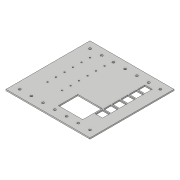
# Autodesk Inventor part: panel
Saved by Autodesk Inventor 2017 (Build 210142000, 142)
## iProperties
Created: 2016-07-20
Part Number: panel
Material: Generic
Document SubType Name: Modeling
Designer: Zuhra Abdurashidova
Density: 1 g/cm^3
Appearance: Default
Author: Zuhra Abdurashidova
Autodesk Inventor part; units mm, degrees
ref_plane "YZ Plane" through (0, 0, 0) normal (1, 0, 0) x (0, 1, 0)
ref_plane "XZ Plane" through (0, 0, 0) normal (0, 1, 0) x (-1, 0, 0)
ref_plane "XY Plane" through (0, 0, 0) normal (0, 0, 1) x (1, 0, 0)
sketch "Sketch1" plane through (0, 0, 0) normal (0, 1, 0) x (-1, 0, 0)
  line L0 (0, 0) -> (-440, 0)
  line L1 (-440, 0) -> (-440, -440)
  line L2 (-440, -440) -> (0, -440)
  line L3 (0, -440) -> (0, 0)
  line L4 (-73.0377, -365.3) -> (-73.0377, -362.3)
  arc A0 (-73.0377, -362.3) -> (-73.0377, -365.3) centre (-76.2, -363.8) ccw
  line L5 (-149.2377, -365.3) -> (-149.2377, -362.3)
  arc A1 (-149.2377, -362.3) -> (-149.2377, -365.3) centre (-152.4, -363.8) ccw
  line L6 (-73.0377, -320.85) -> (-73.0377, -317.85)
  arc A2 (-73.0377, -317.85) -> (-73.0377, -320.85) centre (-76.2, -319.35) ccw
  line L7 (-149.2377, -320.85) -> (-149.2377, -317.85)
  arc A3 (-149.2377, -317.85) -> (-149.2377, -320.85) centre (-152.4, -319.35) ccw
  line L8 (-73.0377, -276.4) -> (-73.0377, -273.4)
  arc A4 (-73.0377, -273.4) -> (-73.0377, -276.4) centre (-76.2, -274.9) ccw
  line L9 (-149.2377, -276.4) -> (-149.2377, -273.4)
  arc A5 (-149.2377, -273.4) -> (-149.2377, -276.4) centre (-152.4, -274.9) ccw
  line L10 (-73.0377, -231.95) -> (-73.0377, -228.95)
  arc A6 (-73.0377, -228.95) -> (-73.0377, -231.95) centre (-76.2, -230.45) ccw
  line L11 (-149.2377, -231.95) -> (-149.2377, -228.95)
  arc A7 (-149.2377, -228.95) -> (-149.2377, -231.95) centre (-152.4, -230.45) ccw
  line L12 (-73.0377, -187.5) -> (-73.0377, -184.5)
  arc A8 (-73.0377, -184.5) -> (-73.0377, -187.5) centre (-76.2, -186) ccw
  line L13 (-149.2377, -187.5) -> (-149.2377, -184.5)
  arc A9 (-149.2377, -184.5) -> (-149.2377, -187.5) centre (-152.4, -186) ccw
  line L14 (-73.0377, -143.05) -> (-73.0377, -140.05)
  arc A10 (-73.0377, -140.05) -> (-73.0377, -143.05) centre (-76.2, -141.55) ccw
  line L15 (-149.2377, -143.05) -> (-149.2377, -140.05)
  arc A11 (-149.2377, -140.05) -> (-149.2377, -143.05) centre (-152.4, -141.55) ccw
  line L16 (-344.75, -344.75) -> (-382.85, -344.75)
  line L17 (-382.85, -344.75) -> (-382.85, -382.85)
  line L18 (-382.85, -382.85) -> (-344.75, -382.85)
  line L19 (-344.75, -382.85) -> (-344.75, -344.75)
  line L20 (-344.75, -344.75) -> (-382.85, -382.85) construction
  line L21 (-382.85, -344.75) -> (-344.75, -382.85) construction
  line L22 (-344.75, -300.3) -> (-382.85, -300.3)
  line L23 (-344.75, -338.4) -> (-344.75, -300.3)
  line L24 (-382.85, -300.3) -> (-382.85, -338.4)
  line L25 (-382.85, -338.4) -> (-344.75, -338.4)
  line L26 (-382.85, -300.3) -> (-344.75, -338.4) construction
  line L27 (-344.75, -300.3) -> (-382.85, -338.4) construction
  line L28 (-344.75, -255.85) -> (-382.85, -255.85)
  line L29 (-344.75, -293.95) -> (-344.75, -255.85)
  line L30 (-382.85, -255.85) -> (-382.85, -293.95)
  line L31 (-382.85, -293.95) -> (-344.75, -293.95)
  line L32 (-382.85, -255.85) -> (-344.75, -293.95) construction
  line L33 (-344.75, -255.85) -> (-382.85, -293.95) construction
  line L34 (-344.75, -211.4) -> (-382.85, -211.4)
  line L35 (-344.75, -249.5) -> (-344.75, -211.4)
  line L36 (-382.85, -211.4) -> (-382.85, -249.5)
  line L37 (-382.85, -249.5) -> (-344.75, -249.5)
  line L38 (-382.85, -211.4) -> (-344.75, -249.5) construction
  line L39 (-344.75, -211.4) -> (-382.85, -249.5) construction
  line L40 (-344.75, -166.95) -> (-382.85, -166.95)
  line L41 (-344.75, -205.05) -> (-344.75, -166.95)
  line L42 (-382.85, -166.95) -> (-382.85, -205.05)
  line L43 (-382.85, -205.05) -> (-344.75, -205.05)
  line L44 (-382.85, -166.95) -> (-344.75, -205.05) construction
  line L45 (-344.75, -166.95) -> (-382.85, -205.05) construction
  line L46 (-344.75, -122.5) -> (-382.85, -122.5)
  line L47 (-344.75, -160.6) -> (-344.75, -122.5)
  line L48 (-382.85, -122.5) -> (-382.85, -160.6)
  line L49 (-382.85, -160.6) -> (-344.75, -160.6)
  line L50 (-382.85, -122.5) -> (-344.75, -160.6) construction
  line L51 (-344.75, -122.5) -> (-382.85, -160.6) construction
  line L52 (-211.4, -165.1) -> (-338.4, -165.1)
  line L53 (-338.4, -165.1) -> (-338.4, -63.5)
  line L54 (-338.4, -63.5) -> (-211.4, -63.5)
  line L55 (-211.4, -63.5) -> (-211.4, -165.1)
  point P0 (-363.8, -363.8)
  point P1 (-363.8, -319.35)
  point P2 (-363.8, -274.9)
  point P3 (-363.8, -230.45)
  point P4 (-363.8, -186)
  point P5 (-363.8, -141.55)
  dimension "d0" = 440
  dimension "d1" = 440
  dimension "d107" = 3.5
  dimension "d109" = 3
  dimension "d111" = 76.2
  dimension "d135" = 76.2
  dimension "d138" = 76.2
  dimension "d141" = 44.45
  dimension "d144" = 38.1
  dimension "d145" = 38.1
  dimension "d146" = 76.2
  dimension "d147" = 76.2
  dimension "d150" = 44.45
  dimension "d155" = 101.6
  dimension "d156" = 127
  dimension "d157" = 101.6
  dimension "d158" = 63.5
  constraints: 112 end point, 24 point on circle, 12 centre point, 12 midpoint, 6 parallel, 4 horizontal, 3 perpendicular, 3 vertical, 110 other
  measures "d0" distance of L1.end L2.end
  measures "d1" distance of L0.end L1.end
  measures "d107" radius of A0
  measures "d109" distance of L4.start L4.end
  measures "d111" distance from line of L2 A0.centre
  measures "d135" distance from line of A0.centre L3
  measures "d138" distance of L4.start L5.start
  measures "d141" distance of L4.start L6.start
  measures "d144" distance of L17.end L18.end
  measures "d145" distance of L16.end L17.end
  measures "d146" distance from line of L2 point (-363.8, -363.8)
  measures "d147" distance from line of L1 point (-363.8, -363.8)
  measures "d150" distance of L16.start L22.start
  measures "d155" distance of L52.end L53.end
  measures "d156" distance of L52.start L52.end
  measures "d157" distance between parallel lines of L53 L1
  measures "d158" distance between parallel lines of L54 L0
extrude "panel body" add sketch "Sketch1" along normal blind 6.35
sketch "Sketch2" plane through (0, 6.35, 0) normal (0, 1, 0) x (1, 0, 0)
  line L0 (35.95, 35.95) -> (404.05, 35.95) construction
  line L1 (404.05, 35.95) -> (404.05, 404.05) construction
  line L2 (404.05, 404.05) -> (35.95, 404.05) construction
  line L3 (35.95, 404.05) -> (35.95, 35.95) construction
  line L4 (35.95, 35.95) -> (404.05, 404.05) construction
  line L5 (404.05, 35.95) -> (35.95, 404.05) construction
  line L6 (440, 440) -> (0, 440) projected
  line L7 (220, 440) -> (220, 3.9535) construction
  line L8 (0, 440) -> (0, 0) projected
  line L9 (0, 220) -> (440, 220) construction
  line L10 (440, 0) -> (440, 440) projected
  circle A0 centre (35.95, 404.05) radius 6
  circle A1 centre (97.3, 404.05) radius 6
  circle A2 centre (158.65, 404.05) radius 6
  circle A3 centre (220, 404.05) radius 6
  circle A4 centre (281.35, 404.05) radius 6
  circle A5 centre (342.7, 404.05) radius 6
  circle A6 centre (404.05, 404.05) radius 6
  circle A7 centre (35.95, 35.95) radius 6
  circle A8 centre (158.65, 35.95) radius 6
  circle A9 centre (97.3, 35.95) radius 6
  circle A10 centre (220, 35.95) radius 6
  circle A11 centre (281.35, 35.95) radius 6
  circle A12 centre (342.7, 35.95) radius 6
  circle A13 centre (404.05, 35.95) radius 6
  point P0 (220, 220)
  dimension "d161" = 368.1
  dimension "d162" = 368.1
  dimension "d163" = 12
  dimension "d166" = 61.35
  dimension "d173" = 368.1
  constraints: 16 end point, 14 centre point, 5 midpoint, 2 horizontal, 2 parallel, 2 vertical, 1 coincident, 1 perpendicular, 28 other
  measures "d161" distance of L2.end L1.end
  measures "d162" distance of L1.end L0.end
  measures "d163" diameter of A0
  measures "d166" distance of A0.centre A1.centre
  measures "d173" distance of A0.centre A7.centre
extrude "Extrusion4" cut sketch "Sketch2" against normal up to next
body "Solid3"
